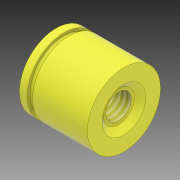
# Autodesk Inventor part: igus_DST-JSRM-1413DS6.35x2.54
Saved by Autodesk Inventor 2017 SP1 (Build 210196100, 196)
## iProperties
Created: 2017-06-12
Part Number: igus_DST-JSRM-1413DS6.35x2.54
Material: Generic
Document SubType Name: Modeling
Designer: Tomasz
Density: 1 g/cm^3
Appearance: Smooth - Yellow
Author: Tomasz
Autodesk Inventor part; units mm, degrees
ref_plane "YZ Plane" through (0, 0, 0) normal (1, 0, 0) x (0, 1, 0)
ref_plane "XZ Plane" through (0, 0, 0) normal (0, 1, 0) x (-1, 0, 0)
ref_plane "XY Plane" through (0, 0, 0) normal (0, 0, 1) x (1, 0, 0)
sketch "Sketch2" plane through (0, 0, 0) normal (0, 0, 1) x (1, 0, 0)
  line L0 (0, 0) -> (18.2937, 0)
  line L1 (0, 4.2) -> (0, 7)
  line L2 (0, 7) -> (1.5, 7)
  line L3 (1.5, 7) -> (1.5, 6.5)
  line L4 (1.5, 6.5) -> (2.5, 6.5)
  line L5 (2.5, 6.5) -> (2.5, 7)
  line L6 (2.5, 7) -> (13, 7)
  line L7 (13, 7) -> (13, 4.2)
  line L8 (0, 4.2) -> (1, 3)
  line L9 (1, 3) -> (1, 0)
  line L10 (13, 4.2) -> (12, 3)
  line L11 (12, 3) -> (12, 0)
  dimension "d12" = 13
  dimension "d13" = 7
  dimension "d14" = 1.5
  dimension "d15" = 1
  dimension "d16" = 0.5
  dimension "d17" = 3
  dimension "d18" = 1
  dimension "d19" = 1.2
  dimension "d20" = 1
  constraints: 24 end point, 7 perpendicular, 5 point on line, 2 horizontal alignment, 1 horizontal, 1 vertical
  measures "d12" distance between parallel lines of L7 L1
  measures "d13" distance from line of L2 L0.start
  measures "d14" distance between parallel lines of L3 L1
  measures "d15" distance between parallel lines of L5 L3
  measures "d16" distance between parallel lines of L4 L2
  measures "d17" distance from line of L8.end L0
  measures "d18" distance from line of L0.start L9
  measures "d19" vertical distance of L8.end L1.start
  measures "d20" distance between parallel lines of L11 L7
revolve "Revolution1" add sketch "Sketch2" angle 360 about axis through (0, 0, 0) along (1, 0, 0)
hole "Hole2" at (1, 0, 0) direction (1, 0, 0) diameter 4.917 end through all thread size "M6x1" class "6H" standard "ANSI Metric M Profile"
body "Solid2"
